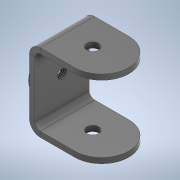
# Autodesk Inventor part: Hinge
Saved by Autodesk Inventor 2020 (Build 240168000, 168)
## iProperties
Created: 2021-07-08
Part Number: Hinge
Material: Steel, Carbon
Document SubType Name: Sheet Metal
Designer: Simon.Alvarez
Density: 7.85 g/cm^3
Sheet Metal Rule: Default_mm
Appearance: Semi-Polished
Author: Simon.Alvarez
Autodesk Inventor part; units mm, degrees
ref_plane "YZ Plane" through (0, 0, 0) normal (1, 0, 0) x (0, 1, 0)
ref_plane "XZ Plane" through (0, 0, 0) normal (0, 1, 0) x (-1, 0, 0)
ref_plane "XY Plane" through (0, 0, 0) normal (0, 0, 1) x (1, 0, 0)
sketch "Sketch1" plane through (0, 0, 0) normal (0, 1, 0) x (-1, 0, 0)
  line L0 (20, 15) -> (-20, 15)
  line L1 (-20, 15) -> (-20, -15)
  line L2 (-20, -15) -> (20, -15)
  line L3 (20, -15) -> (20, 15)
  line L4 (20, 15) -> (-20, -15) construction
  line L5 (-20, 15) -> (20, -15) construction
  point P0 (0, 0)
  dimension "d0" = 40
  dimension "d1" = 30
  constraints: 12 end point, 2 midpoint, 2 parallel, 1 horizontal, 1 perpendicular
  measures "d0" distance of L1.end L2.end
  measures "d1" distance of L0.end L1.end
extrude "Extrusion1" add sketch "Sketch1" along normal blind 3
sketch "Sketch2" plane through (-17, 3, -15) normal (-1, 0, 0) x (0, -1, 0)
  line L0 (0, 30) -> (0, 0)
  line L1 (0, 0) -> (43, 0)
  line L2 (43, 0) -> (43, 30)
  line L3 (43, 30) -> (0, 30)
  constraints: 6 end point, 1 horizontal, 1 perpendicular, 1 vertical
edge flange "Flange1" height 43 angle 90 thickness 3 bend radius 3 thickness toward (-1, 0, 0) relief tear relief width 3 relief depth 1.5 edges at (-20, 0, 0) wall of the first edge with corners at (-17, 3, 15) (-17, 3, -15) (-17, -40, -15) (-17, -40, 15)
bend "Bend1"
corner "Corner1"
sketch "Sketch3" plane through (-20, -37, -15) normal (0, -1, 0) x (1, 0, 0)
  line L0 (0, 30) -> (0, 0)
  line L1 (0, 0) -> (40, 0)
  line L2 (40, 0) -> (40, 30)
  line L3 (40, 30) -> (0, 30)
  constraints: 6 end point, 1 horizontal, 1 perpendicular, 1 vertical
edge flange "Flange2" height 40 angle 90 thickness 3 bend radius 3 thickness toward (0, -1, 0) relief tear relief width 3 relief depth 1.5 edges at (-17, -40, 0) wall of the first edge with corners at (-20, -37, 15) (-20, -37, -15) (20, -37, -15) (20, -37, 15)
bend "Bend2"
corner "Corner2"
fillet "Fillet1" radius 15 4 edges at (20, 1.5, 15) (20, 1.5, -15) (20, -38.5, -15) (20, -38.5, 15)
sketch "Sketch4" plane through (0, 3, 0) normal (0, 1, 0) x (1, 0, 0)
  point P0 (0, 0)
  point P1 (0, 0)
  constraints: 1 coincident
hole "Hole1" at (0, 3, 0) direction (0, -1, 0) diameter 6.6 end through all clearance for "Flat Head Machine Screw" size "M6" standard "Ansi Metric M Profile"
sketch "Sketch5" plane through (-20, -3, -15) normal (-1, 0, 0) x (0, 0, 1)
  line L0 (0, 0) -> (0, -31) projected
  line L1 (0, -15.5) -> (30, -15.5)
  line L2 (30, 0) -> (30, -31) projected
  point P0 (15, 3)
  point P1 (15, -15.5)
  constraints: 3 midpoint, 2 end point
hole "Hole2" at (-20, -18.5, 0) direction (1, 0, 0) diameter 4.917 end through all thread size "M6x1" class "6H" standard "ANSI Metric M Profile"
sketch "Sketch6" plane through (-20, -3, -15) normal (-1, 0, 0) x (0, 0, 1)
  circle A0 centre (15, -15.5) radius 2.4585 projected
  circle A1 centre (15, -15.5) radius 10
  circle A2 centre (15, -15.5) radius 12.5
  point P0 (15, 3)
  dimension "d40" = 20
  dimension "d42" = 25
  constraints: 2 centre point, 1 coincident
  measures "d40" diameter of A1
  measures "d42" diameter of A2
extrude "Extrusion2" add sketch "Sketch6" along normal blind 3 contours A2
fillet "Fillet2" radius 1 1 edges at (-20, -18.5, -12.5)
fillet "Fillet3" radius 1 1 edges at (-20, -18.5, -10)
equation "\"d31\" = Thickness"
equation "\"d4\" = Thickness"
equation "\"d5\" = BendReliefWidth"
equation "\"d6\" = BendReliefDepth"
equation "\"d7\" = MinimumRemnant"
equation "\"d8\" = TransitionRadius"
equation "\"d11\" = BendRadius"
equation "\"d12\" = CornerReliefSize"
equation "\"d13\" = GapSize"
equation "\"d14\" = JacobiRadiusSize"
equation "\"d15\" = BendReliefWidth"
equation "\"d16\" = BendReliefDepth"
equation "\"d17\" = MinimumRemnant"
equation "\"d18\" = TransitionRadius"
equation "\"d21\" = BendRadius"
equation "\"d22\" = CornerReliefSize"
equation "\"d23\" = GapSize"
equation "\"d24\" = JacobiRadiusSize"
equation "\"BendRadius\" = Thickness"
equation "\"BendReliefWidth\" = Thickness"
equation "\"BendReliefDepth\" = 0.5 * Thickness"
equation "\"CornerReliefSize\" = 4 * Thickness"
equation "\"MinimumRemnant\" = 2 * Thickness"
equation "\"TransitionRadius\" = BendRadius"
equation "\"JacobiRadiusSize\" = BendRadius"
equation "\"GapSize\" = Thickness"
equation "\"Thickness\" = 3"
body "Solid1"
